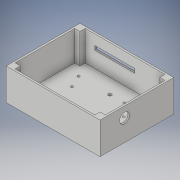
# Autodesk Inventor part: 546-1590BBS-Pi
Saved by Autodesk Inventor 2018 (Build 220112000, 112)
## iProperties
Created: 2018-04-27
Part Number: 546-1590BBS-Pi
Material: Generic
Document SubType Name: Modeling
Designer: bbramman
Density: 1 g/cm^3
Appearance: Default
Author: bbramman
Autodesk Inventor part; units mm, degrees
ref_plane "YZ Plane" through (0, 0, 0) normal (1, 0, 0) x (0, 1, 0)
ref_plane "XZ Plane" through (0, 0, 0) normal (0, 1, 0) x (-1, 0, 0)
ref_plane "XY Plane" through (0, 0, 0) normal (0, 0, 1) x (1, 0, 0)
sketch "Sketch1" plane through (0, 0, 0) normal (0, 1, 0) x (-1, 0, 0)
  line L0 (-59.7535, -47.0027) -> (59.7535, -47.0027)
  line L1 (59.7535, -47.0027) -> (59.7535, 47.0027)
  line L2 (59.7535, 47.0027) -> (-59.7535, 47.0027)
  line L3 (-59.7535, 47.0027) -> (-59.7535, -47.0027)
  line L4 (-59.7535, -47.0027) -> (59.7535, 47.0027) construction
  line L5 (59.7535, -47.0027) -> (-59.7535, 47.0027) construction
  point P0 (0, 0)
  dimension "d0" = 119.507
  dimension "d1" = 94.0054
  constraints: 12 end point, 2 midpoint, 2 parallel, 1 horizontal, 1 perpendicular
  measures "d0" distance of L2.end L1.end
  measures "d1" distance of L1.end L0.end
extrude "Extrusion1" add sketch "Sketch1" along normal mid plane 2.2606
sketch "Sketch2" plane through (0, 1.1303, 0) normal (0, 1, 0) x (1, 0, 0)
  line L0 (-59.7535, 47.0027) -> (-59.7535, -47.0027) projected
  line L1 (59.7535, -47.0027) -> (59.7535, 47.0027) projected
  line L2 (-59.7535, -47.0027) -> (59.7535, -47.0027)
  line L3 (59.7535, -47.0027) -> (59.7535, 47.0027)
  line L4 (59.7535, 47.0027) -> (-59.7535, 47.0027)
  line L5 (-59.7535, 47.0027) -> (-59.7535, -47.0027)
  line L6 (57.4929, -44.7421) -> (-57.4929, 44.7421) construction
  line L7 (-57.4929, -44.7421) -> (57.4929, 44.7421) construction
  line L8 (-59.7535, -47.0027) -> (59.7535, -47.0027) projected
  line L9 (-59.7535, -47.0027) -> (-50.7619, -47.0027)
  line L10 (-59.7535, -38.0111) -> (-59.7535, -47.0027)
  line L11 (-59.7535, 47.0027) -> (-50.7619, 47.0027)
  line L12 (-59.7535, 38.0111) -> (-59.7535, 47.0027)
  line L13 (59.7535, 47.0027) -> (-59.7535, 47.0027) projected
  line L14 (59.7535, 47.0027) -> (50.7619, 47.0027)
  line L15 (59.7535, 38.0111) -> (59.7535, 47.0027)
  line L16 (59.7535, -47.0027) -> (50.7619, -47.0027)
  line L17 (59.7535, -38.0111) -> (59.7535, -47.0027)
  line L18 (-50.7619, -44.7421) -> (-50.7619, -38.0111)
  line L19 (-50.7619, -38.0111) -> (-57.4929, -38.0111)
  line L20 (-57.4929, 38.0111) -> (-50.7619, 38.0111)
  line L21 (-50.7619, 38.0111) -> (-50.7619, 44.7421)
  line L22 (50.7619, 38.0111) -> (57.4929, 38.0111)
  line L23 (50.7619, 44.7421) -> (50.7619, 38.0111)
  line L24 (57.4929, -38.0111) -> (50.7619, -38.0111)
  line L25 (50.7619, -38.0111) -> (50.7619, -44.7421)
  line L26 (-50.7619, -44.7421) -> (50.7619, -44.7421)
  line L27 (57.4929, -38.0111) -> (57.4929, 38.0111)
  line L28 (50.7619, 44.7421) -> (-50.7619, 44.7421)
  line L29 (-57.4929, 38.0111) -> (-57.4929, -38.0111)
  point P0 (0, 0)
  dimension "d4" = 114.9858
  dimension "d5" = 89.4842
  dimension "d6" = 8.9916
  dimension "d7" = 8.9916
  dimension "d10" = 8.9916
  dimension "d11" = 8.9916
  constraints: 52 end point, 7 horizontal, 3 perpendicular, 2 midpoint, 2 parallel
  measures "d4" distance of L6.end L7.end
  measures "d5" distance of L7.start L6.end
  measures "d6" distance of L10.start L18.end
  measures "d7" distance of L18.end L9.end
  measures "d10" distance of L15.start L22.start
  measures "d11" distance of L22.start L14.end
extrude "Extrusion2" add sketch "Sketch2" along normal blind 38.1
sketch "Sketch3" plane through (0, 1.1303, 0) normal (0, 1, 0) x (1, 0, 0)
  circle A0 centre (0, -25.4) radius 2.0828
  circle A1 centre (0, 25.4) radius 2.0828
  point P0 (0, 0)
  dimension "d18" = 4.1656
  dimension "d19" = 4.1656
  constraints: 2 centre point
  measures "d18" diameter of A0
  measures "d19" diameter of A1
extrude "Extrusion3" cut sketch "Sketch3" against normal through all
sketch "Sketch4" plane through (0, 1.1303, 0) normal (0, 1, 0) x (1, 0, 0)
  line L0 (43.434, -28.8417) -> (-43.434, 28.8417) construction
  line L1 (-43.434, -28.8417) -> (43.434, 28.8417) construction
  line L2 (32.9946, -9.9949) -> (-32.9946, 9.9949) construction
  line L3 (-32.9946, -9.9949) -> (32.9946, 9.9949) construction
  circle A0 centre (-40.259, -25.6667) radius 1.4224
  circle A1 centre (-40.259, 25.6667) radius 1.4224
  circle A2 centre (18.034, -25.6667) radius 1.4224
  circle A3 centre (18.034, 25.6667) radius 1.4224
  circle A4 centre (-32.9946, -9.9949) radius 1.4986
  circle A5 centre (-32.9946, 9.9949) radius 1.4986
  circle A6 centre (32.9946, 9.9949) radius 1.4986
  circle A7 centre (32.9946, -9.9949) radius 1.4986
  point P0 (0, 0)
  point P1 (0, 0)
  dimension "d22" = 86.868
  dimension "d23" = 57.6834
  dimension "d25" = 19.9898
  dimension "d30" = 2.8448
  dimension "d31" = 2.8448
  dimension "d36" = 2.8448
  dimension "d37" = 2.8448
  dimension "d38" = 2.9972
  dimension "d39" = 2.9972
  dimension "d40" = 2.9972
  dimension "d41" = 2.9972
  constraints: 8 centre point, 8 end point, 6 midpoint, 4 coincident
  measures "d22" distance of L0.end L1.end
  measures "d23" distance of L1.start L0.end
  measures "d25" distance of L3.start L2.end
  measures "d30" diameter of A0
  measures "d31" diameter of A1
  measures "d36" diameter of A2
  measures "d37" diameter of A3
  measures "d38" diameter of A4
  measures "d39" diameter of A5
  measures "d40" diameter of A6
  measures "d41" diameter of A7
extrude "Extrusion4" cut sketch "Sketch4" against normal through all
sketch "Sketch6" plane through (57.4929, 1.1303, -38.0111) normal (-1, 0, 0) x (0, 0, 1)
  circle A0 centre (53.7096, 24.7973) radius 6.35
  point P0 (38.0111, -1.1303)
  dimension "d44" = 12.7
  constraints: 1 centre point
  measures "d44" diameter of A0
extrude "Extrusion5" cut sketch "Sketch6" against normal through all
sketch "Sketch7" plane through (-50.7619, 1.1303, -44.7421) normal (0, 0, 1) x (1, 0, 0)
  line L0 (12.3731, 25.4) -> (63.1731, 25.4)
  line L1 (63.1731, 25.4) -> (63.1731, 20.2873)
  line L2 (63.1731, 20.2873) -> (12.3731, 20.2873)
  line L3 (12.3731, 20.2873) -> (12.3731, 25.4)
  point P0 (50.7619, -1.1303)
  dimension "d47" = 50.8
  constraints: 8 end point, 2 parallel, 1 horizontal, 1 perpendicular
  measures "d47" distance of L1.end L2.end
extrude "Extrusion6" cut sketch "Sketch7" against normal through all
body "Solid1"
